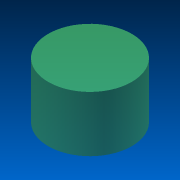
# Autodesk Inventor part: GoPro Hero 3 Indicator Cover
Saved by Autodesk Inventor 2015 (Build 190159000, 159)
## iProperties
Created: 2013-02-18
Material: Glass, Frosted
Document SubType Name: Modeling
Designer: sdarley
Density: 1 g/cm^3
Project: GoPro Hero 3 HD Camera
Description: GoPro Hero 3 Indicator Cover
Appearance: Frosted(1)
Author: sdarley
Title: GoPro Hero 3 Indicator Cover
Revision Number: 1
Autodesk Inventor part; units mm, degrees
ref_plane "YZ Plane" through (0, 0, 0) normal (1, 0, 0) x (0, 1, 0)
ref_plane "XZ Plane" through (0, 0, 0) normal (0, 1, 0) x (-1, 0, 0)
ref_plane "XY Plane" through (0, 0, 0) normal (0, 0, 1) x (1, 0, 0)
sketch "Sketch1" plane through (0, 0, 0) normal (0, 0, 1) x (1, 0, 0)
  circle A0 centre (0, 0) radius 1.5
  dimension "d0" = 3
  constraints: 1 centre point, 1 coincident
  measures "d0" diameter of A0
extrude "Extrusion1" add sketch "Sketch1" along normal blind 2
body "Solid1"
